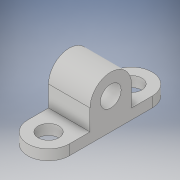
# Autodesk Inventor part: Tarea 1 - Melany Escobar
Saved by Autodesk Inventor 2019.1 (Build 231200000, 200)
## iProperties
Created: 2024-02-03
Part Number: Tarea 1 - Melany Escobar
Material: Generic
Document SubType Name: Modeling
Designer: clariheelen
Density: 1 g/cm^3
Appearance: Default
Author: clariheelen
Autodesk Inventor part; units mm, degrees
ref_plane "YZ Plane" through (0, 0, 0) normal (1, 0, 0) x (0, 1, 0)
ref_plane "XZ Plane" through (0, 0, 0) normal (0, 1, 0) x (-1, 0, 0)
ref_plane "XY Plane" through (0, 0, 0) normal (0, 0, 1) x (1, 0, 0)
sketch "Sketch1" plane through (0, 0, 0) normal (0, 1, 0) x (-1, 0, 0)
  line L0 (0, 40) -> (0, -40) construction
  line L1 (-20, 40) -> (-20, -40)
  line L2 (20, -40) -> (20, 40)
  arc A0 (20, 40) -> (-20, 40) centre (0, 40) ccw
  arc A1 (-20, -40) -> (20, -40) centre (0, -40) ccw
  point P0 (0, 0)
  dimension "d0" = 40
  dimension "d1" = 40
  constraints: 8 end point, 4 point on circle, 4 tangent, 2 centre point, 1 midpoint, 1 parallel, 1 vertical
  measures "d0" distance of point (0, 0) L0.end
  measures "d1" diameter of A1
extrude "Extrusion1" add sketch "Sketch1" along normal blind 10
sketch "Sketch2" plane through (0, 10, 0) normal (0, 1, 0) x (1, 0, 0)
  line L0 (20, -40) -> (20, 40) projected
  line L1 (-20, -20) -> (20, -20)
  line L2 (20, -20) -> (20, 20)
  line L3 (20, 20) -> (-20, 20)
  line L4 (-20, 20) -> (-20, -20)
  line L5 (-20, -20) -> (20, 20) construction
  line L6 (20, -20) -> (-20, 20) construction
  point P0 (0, 0)
  constraints: 12 end point, 2 midpoint, 2 parallel, 1 horizontal, 1 perpendicular, 1 point on line
extrude "Extrusion2" add sketch "Sketch2" along normal blind 20
sketch "Sketch3" plane through (20, 0, 40) normal (1, 0, 0) x (0, 0, -1)
  line L0 (20, 30) -> (60, 30) projected
  circle A0 centre (40, 30) radius 20
  point P0 (40, 0)
  constraints: 1 horizontal alignment, 1 midpoint, 2 other
extrude "Extrusion3" add sketch "Sketch3" against normal blind 40
sketch "Sketch4" plane through (0, 10, 0) normal (0, 1, 0) x (1, 0, 0)
  arc A0 (-20, -40) -> (20, -40) centre (0, -40) ccw projected
  circle A1 centre (0, -40) radius 10
  arc A2 (20, 40) -> (-20, 40) centre (0, 40) ccw projected
  circle A3 centre (0, 40) radius 10
  point P0 (0, 0)
  dimension "d9" = 20
  dimension "d10" = 20
  constraints: 2 centre point, 2 coincident
  measures "d9" diameter of A1
  measures "d10" diameter of A3
extrude "Extrusion4" cut sketch "Sketch4" against normal blind 10 contours A1
sketch "Sketch5" plane through (0, 10, 0) normal (0, 1, 0) x (1, 0, 0)
  arc A0 (20, 40) -> (-20, 40) centre (0, 40) ccw projected
  circle A1 centre (0, 40) radius 10
  point P0 (0, 0)
  dimension "d13" = 20
  constraints: 1 centre point, 1 coincident
  measures "d13" diameter of A1
extrude "Extrusion5" cut sketch "Sketch5" against normal blind 10
sketch "Sketch6" plane through (20, 0, 40) normal (1, 0, 0) x (0, 0, -1)
  arc A0 (60, 30) -> (20, 30) centre (40, 30) ccw projected
  circle A1 centre (40, 30) radius 10
  point P0 (40, 0)
  dimension "d16" = 20
  constraints: 1 centre point, 1 coincident
  measures "d16" diameter of A1
extrude "Extrusion6" cut sketch "Sketch6" against normal blind 40
body "Solid1"
